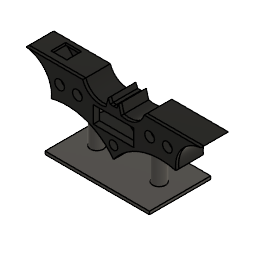
Bat Clock (Autodesk Fusion 360 design; units mm, degrees)
part number: 2025-11-05-17-47-18-195
part number: 2025-11-05-18-19-24-165
part number: 2025-11-05-18-19-49-827
part number: 2025-11-05-19-01-45-549
Autodesk Fusion 360 part; units mm, degrees
sketch "Sketch1" plane through (0, 0, 0) normal (0, 0, 1) x (1, 0, 0)
  line L0 (0, 0) -> (70.0024, 0)
  line L1 (0, 0) -> (0, -40.005)
  dimension "d1" = 70.0024
  dimension "d2" = 40.005
  constraint coincident L0.start L1.start
  constraint horizontal L0
  constraint perpendicular L0 L1
  measures "d1" distance of L0.start L0.end
  measures "d2" distance of L0.start L1.end
sketch "Sketch2" plane through (0, 0, 0) normal (0, 0, 1) x (1, 0, 0)
  line L0 (0, 0) -> (0, -40.64)
  arc A0 (0, -38.1) -> (-51.5436, -20.32) centre (-38.6745, -66.6145) ccw
  arc A1 (-51.5436, -20.32) -> (-72.3189, 6.443) centre (-75.1219, -17.178) ccw
  line L1 (-72.3189, 6.443) -> (-25.4, 6.443)
  arc A2 (-25.4, 6.443) -> (-6.3115, -3.5502) centre (-10.7993, 11.1049) ccw
  line L2 (-6.3115, -3.5502) -> (-4.3391, 3.8132)
  line L3 (-4.3391, 3.8132) -> (-2.7613, 0.1315)
  line L4 (-2.7613, 0.1315) -> (0, 0)
  arc A3 (51.5436, -20.32) -> (0, -38.1) centre (38.6745, -66.6145) ccw
  line L5 (4.3391, 3.8132) -> (2.7613, 0.1315)
  line L6 (72.3189, 6.443) -> (25.4, 6.443)
  arc A4 (6.3115, -3.5502) -> (25.4, 6.443) centre (10.7993, 11.1049) ccw
  line L7 (2.7613, 0.1315) -> (0, 0)
  arc A5 (72.3189, 6.443) -> (51.5436, -20.32) centre (75.1219, -17.178) ccw
  line L8 (6.3115, -3.5502) -> (4.3391, 3.8132)
  constraint coincident L0.start L4.end
  constraint vertical L0
  constraint coincident L0 A0.start
  constraint horizontal L1
  constraint symmetric L0 A0.start A3.end
  constraint symmetric L0 A0.end A3.start
  constraint symmetric L0 A0 A3
  constraint symmetric L0 A1.end L6.start
  constraint symmetric L0 A1 A5
  constraint symmetric L0 L1.end L6.end
  constraint symmetric L0 A2.end A4.start
  constraint symmetric L0 A2 A4
  constraint symmetric L0 L2.end L5.start
  constraint symmetric L0 L3.end L5.end
  constraint symmetric L0 L4.end L7.end
extrude "Extrude1" add sketch "Sketch2" along normal blind 20.32 makes body 1
shell "Shell1" thickness 2.032 removed faces 1 at (39.0183, -7.033, 20.32) on bodies 1
sketch "Sketch4" plane through (0, 0, 20.32) normal (0, 0, 1) x (-1, 0, 0)
  arc A0 (-60.9613, -4.411) -> (-49.308, 17.6745) centre (-75.1219, 17.178) ccw
  arc A1 (-49.308, 17.6745) -> (0, 34.795) centre (-38.6745, 66.6145) ccw
  arc A2 (0, 34.795) -> (49.308, 17.6745) centre (38.6745, 66.6145) ccw
  arc A3 (49.308, 17.6745) -> (60.9613, -4.411) centre (75.1219, 17.178) ccw
  line L0 (60.9613, -4.411) -> (26.8156, -4.411)
  arc A4 (26.8156, -4.411) -> (4.6283, 5.1201) centre (10.7993, -11.1049) ccw
  line L1 (4.6283, 5.1201) -> (3.7539, 1.8555)
  line L2 (3.7539, 1.8555) -> (0, 2.0343)
  line L3 (0, 2.0343) -> (-3.7539, 1.8555)
  line L4 (-3.7539, 1.8555) -> (-4.6283, 5.1201)
  arc A5 (-4.6283, 5.1201) -> (-26.8156, -4.411) centre (-10.7993, -11.1049) ccw
  line L5 (-26.8156, -4.411) -> (-60.9613, -4.411)
  line L6 (-72.3189, -6.443) -> (-25.4, -6.443)
  arc A6 (-6.3115, 3.5502) -> (-25.4, -6.443) centre (-10.7993, -11.1049) ccw
  line L7 (-6.3115, 3.5502) -> (-4.3391, -3.8132)
  line L8 (-4.3391, -3.8132) -> (-2.7613, -0.1315)
  line L9 (-2.7613, -0.1315) -> (0, 0)
  line L10 (0, 0) -> (2.7613, -0.1315)
  line L11 (2.7613, -0.1315) -> (4.3391, -3.8132)
  line L12 (4.3391, -3.8132) -> (6.3115, 3.5502)
  arc A7 (25.4, -6.443) -> (6.3115, 3.5502) centre (10.7993, -11.1049) ccw
  line L13 (25.4, -6.443) -> (72.3189, -6.443)
  arc A8 (51.5436, 20.32) -> (72.3189, -6.443) centre (75.1219, 17.178) ccw
  arc A9 (0, 38.1) -> (51.5436, 20.32) centre (38.6745, 66.6145) ccw
  arc A10 (-51.5436, 20.32) -> (0, 38.1) centre (-38.6745, 66.6145) ccw
  arc A11 (-72.3189, -6.443) -> (-51.5436, 20.32) centre (-75.1219, 17.178) ccw
sketch "Sketch5" plane through (0, 0, 20.32) normal (0, 0, 1) x (-1, 0, 0)
  arc A0 (-60.9613, -4.411) -> (-49.308, 17.6745) centre (-75.1219, 17.178) ccw
  arc A1 (-49.308, 17.6745) -> (0, 34.795) centre (-38.6745, 66.6145) ccw
  arc A2 (0, 34.795) -> (49.308, 17.6745) centre (38.6745, 66.6145) ccw
  arc A3 (49.308, 17.6745) -> (60.9613, -4.411) centre (75.1219, 17.178) ccw
  line L0 (60.9613, -4.411) -> (26.8156, -4.411)
  arc A4 (26.8156, -4.411) -> (4.6283, 5.1201) centre (10.7993, -11.1049) ccw
  line L1 (4.6283, 5.1201) -> (3.7539, 1.8555)
  line L2 (3.7539, 1.8555) -> (0, 2.0343)
  line L3 (0, 2.0343) -> (-3.7539, 1.8555)
  line L4 (-3.7539, 1.8555) -> (-4.6283, 5.1201)
  arc A5 (-4.6283, 5.1201) -> (-26.8156, -4.411) centre (-10.7993, -11.1049) ccw
  line L5 (-26.8156, -4.411) -> (-60.9613, -4.411)
  line L6 (-72.3189, -6.443) -> (-25.4, -6.443)
  arc A6 (-6.3115, 3.5502) -> (-25.4, -6.443) centre (-10.7993, -11.1049) ccw
  line L7 (-6.3115, 3.5502) -> (-4.3391, -3.8132)
  line L8 (-4.3391, -3.8132) -> (-2.7613, -0.1315)
  line L9 (-2.7613, -0.1315) -> (0, 0)
  line L10 (0, 0) -> (2.7613, -0.1315)
  line L11 (2.7613, -0.1315) -> (4.3391, -3.8132)
  line L12 (4.3391, -3.8132) -> (6.3115, 3.5502)
  arc A7 (25.4, -6.443) -> (6.3115, 3.5502) centre (10.7993, -11.1049) ccw
  line L13 (25.4, -6.443) -> (72.3189, -6.443)
  arc A8 (51.5436, 20.32) -> (72.3189, -6.443) centre (75.1219, 17.178) ccw
  arc A9 (0, 38.1) -> (51.5436, 20.32) centre (38.6745, 66.6145) ccw
  arc A10 (-51.5436, 20.32) -> (0, 38.1) centre (-38.6745, 66.6145) ccw
  arc A11 (-72.3189, -6.443) -> (-51.5436, 20.32) centre (-75.1219, 17.178) ccw
extrude "Extrude3" add sketch "Sketch5" against normal blind 2.54 separate body contours A0 A1 A2 A3 L0 A4 L1 L2 L3 L4 A5 L5 makes body 2
extrude "Extrude4" add sketch "Sketch5" along normal blind 2.54 contours A0 A1 A2 A3 L0 A4 L1 L2 L3 L4 A5 L5 | L6 A6 L7 L8 L9 L10 L11 L12 A7 L13 A8 A9 A10 A11 bodies 2
copy_body "Body->Comp1" bodies 1 removing the originals makes body 3 in component "Body"
copy_body "Body->Comp2" bodies 2 removing the originals makes body 4 in component "Lid"
sketch "Sketch6" plane through (0, 0, 46.2676) normal (0, 0, 1) x (-1, 0, 0)
  line L0 (-12.6934, 7.182) -> (-10.721, -0.1814)
  line L1 (-10.721, -0.1814) -> (-9.1432, 3.5003)
  line L2 (-9.1432, 3.5003) -> (-6.3819, 3.6318)
  line L3 (-6.3819, 3.6318) -> (-3.6206, 3.5003)
  line L4 (-3.6206, 3.5003) -> (-2.0428, -0.1814)
  line L5 (-2.0428, -0.1814) -> (-0.0704, 7.182)
  arc A0 (19.0181, -2.8112) -> (-0.0704, 7.182) centre (4.4174, -7.4731) ccw
  line L6 (19.0181, -2.8112) -> (65.937, -2.8112)
  arc A1 (45.1617, 23.9518) -> (65.937, -2.8112) centre (68.74, 20.8098) ccw
  arc A2 (-6.3819, 41.7318) -> (45.1617, 23.9518) centre (32.2926, 70.2463) ccw
  arc A3 (-57.9256, 23.9518) -> (-6.3819, 41.7318) centre (-45.0564, 70.2463) ccw
  arc A4 (-78.7008, -2.8112) -> (-57.9256, 23.9518) centre (-81.5038, 20.8098) ccw
  line L7 (-78.7008, -2.8112) -> (-31.7819, -2.8112)
  arc A5 (-12.6934, 7.182) -> (-31.7819, -2.8112) centre (-17.1813, -7.4731) ccw
  line L8 (-23.0838, 24.7751) -> (10.32, 24.7751)
  line L9 (10.32, 24.7751) -> (10.32, 10.785)
  line L10 (10.32, 10.785) -> (-23.0838, 10.785)
  line L11 (-23.0838, 10.785) -> (-23.0838, 24.7751)
  line L12 (-23.0838, 24.7751) -> (10.32, 10.785) construction
  line L13 (10.32, 24.7751) -> (-23.0838, 10.785) construction
  point P0 (-6.3819, 17.78)
  dimension "d14" = 58.42
  dimension "d15" = 58.42
  constraint horizontal L8
  constraint perpendicular L8 L9
  constraint parallel L8 L10
  constraint parallel L9 L11
  constraint coincident L12 P0
  constraint coincident L13 P0
  measures "d14" distance of A4.centre L11
  measures "d15" distance of A1.centre L9
extrude "Extrude1'" cut sketch "Sketch6" against normal blind 17.78 contours L8 L9 L10 L11 sketch seen with x (1, 0, 0) y (0, 1, 0) z (0, 0, 1) at (-6.3819, 3.6318, -23.4076) bodies 4 in component "Lid"
sketch "Sketch7" plane through (0, 0, 22.86) normal (0, 0, 1) x (-1, 0, 0)
  line L0 (16.7019, 21.1433) -> (16.7019, 7.1532)
  line L1 (16.7019, 7.1532) -> (-16.7019, 7.1532)
  line L2 (-16.7019, 7.1532) -> (-16.7019, 21.1433)
  line L3 (-16.7019, 21.1433) -> (16.7019, 21.1433)
  line L4 (-6.3115, 3.5502) -> (-4.3391, -3.8132)
  line L5 (-4.3391, -3.8132) -> (-2.7613, -0.1315)
  line L6 (-2.7613, -0.1315) -> (0, 0)
  line L7 (0, 0) -> (2.7613, -0.1315)
  line L8 (2.7613, -0.1315) -> (4.3391, -3.8132)
  line L9 (4.3391, -3.8132) -> (6.3115, 3.5502)
  arc A0 (25.4, -6.443) -> (6.3115, 3.5502) centre (10.7993, -11.1049) ccw
  line L10 (25.4, -6.443) -> (72.3189, -6.443)
  arc A1 (51.5436, 20.32) -> (72.3189, -6.443) centre (75.1219, 17.178) ccw
  arc A2 (0, 38.1) -> (51.5436, 20.32) centre (38.6745, 66.6145) ccw
  arc A3 (-51.5436, 20.32) -> (0, 38.1) centre (-38.6745, 66.6145) ccw
  arc A4 (-72.3189, -6.443) -> (-51.5436, 20.32) centre (-75.1219, 17.178) ccw
  line L11 (-72.3189, -6.443) -> (-25.4, -6.443)
  arc A5 (-6.3115, 3.5502) -> (-25.4, -6.443) centre (-10.7993, -11.1049) ccw
  circle A6 centre (44.5861, 6.8536) radius 4.0005
  line L12 (0, 0) -> (0, 45.72) construction
  circle A7 centre (29.8835, 6.8536) radius 4.0005
  line L13 (44.5861, 6.8536) -> (56.3321, 6.8536) construction
  line L14 (44.5861, 6.8536) -> (0, 7.1532) construction
  circle A8 centre (-29.8835, 6.8536) radius 4.0005
  circle A9 centre (-44.5861, 6.8536) radius 4.0005
  circle A10 centre (0, 27.94) radius 3.5052
  point P0 (-44.5861, 6.8536)
  point P1 (-44.5861, 6.8536)
  dimension "d22" = 8.001
  dimension "d23" = 7.0104
  constraint coincident L6.end L7.start
  constraint perpendicular L3 L12
  constraint equal A6 A7
  constraint coincident A6.centre L13.start
  constraint horizontal L13
  constraint midpoint L1 L14.end
  constraint horizontal A6.centre A7.centre
  constraint symmetric A6 L12 A9
  constraint symmetric L12 A7 A8
  constraint symmetric L12 A6.centre P1
  constraint coincident L12 A10.centre
  measures "d22" diameter of A6
  measures "d23" diameter of A10
extrude "Extrude2" cut sketch "Sketch7" against normal blind 10.16 contours A6 | A7 | A8 | A9 | A10 bodies 4 in component "Lid"
sketch "Sketch8" plane through (0, 6.443, 0) normal (0, 1, 0) x (-1, 0, 0)
  line L0 (25.4, 0) -> (72.3189, 0)
  line L1 (72.3189, 0) -> (72.3189, 20.32)
  line L2 (72.3189, 20.32) -> (25.4, 20.32)
  line L3 (25.4, 20.32) -> (25.4, 0)
  line L4 (46.1169, 15.3428) -> (59.1217, 15.3428)
  line L5 (59.1217, 15.3428) -> (59.1217, 3.354)
  line L6 (59.1217, 3.354) -> (46.1169, 3.354)
  line L7 (46.1169, 3.354) -> (46.1169, 15.3428)
  dimension "d26" = 13.0048
  dimension "d27" = 11.9888
  constraint horizontal L4
  constraint vertical L5
  constraint horizontal L6
  constraint vertical L7
  measures "d26" distance of L4.start L4.end
  measures "d27" distance of L4.start L6.end
extrude "Extrude1''" cut sketch "Sketch8" against normal blind 2.54 contours L4 L5 L6 L7 bodies 3 in component "Body"
sketch "Sketch9" plane through (0, 0, 0) normal (0, 0, 1) x (1, 0, 0)
  circle A0 centre (-10.4491, 0) radius 5.3128
  line L0 (-36.2174, 10.8533) -> (-36.2174, -9.4667)
  line L1 (15.3263, 10.8533) -> (15.3263, -9.4667) construction
  circle A1 centre (41.1016, 0) radius 5.3128
  point P0 (30.6526, 0)
  dimension "d30" = 25.7683
  dimension "d32" = 25.7753
  dimension "d33" = 51.5436
  constraint symmetric origin L1 P0
  constraint symmetric A0 L1 A1
  measures "d30" distance of A0.centre L0
  measures "d32" distance of A0.centre L1
  measures "d33" distance of L0 L1
extrude "Extrude2'" cut sketch "Sketch9" along normal blind 53.34 sketch seen with x (1, 0, 0) y (0, 0, -1) z (0, 1, 0) at (-15.3263, -69.8065, 10.8533) bodies 3 in component "Body"
extrude "Extrude5" add sketch "Sketch9" along normal blind 33.02 separate body makes body 5 at (46.388, -0.529, 11.0067) makes body 6 at (-5.1627, -0.529, 11.0067)
sketch "Sketch10" plane through (0, 0, 0) normal (0, 0, 1) x (1, 0, 0)
  line L0 (58.42, 25.4) -> (-27.94, 25.4)
  line L1 (-27.94, 25.4) -> (-27.94, -25.4)
  line L2 (-27.94, -25.4) -> (58.42, -25.4)
  line L3 (58.42, -25.4) -> (58.42, 25.4)
  line L4 (58.42, 25.4) -> (-27.94, -25.4) construction
  line L5 (-27.94, 25.4) -> (58.42, -25.4) construction
  point P0 (15.24, 0)
  constraint horizontal L0
  constraint perpendicular L0 L1
  constraint parallel L0 L2
  constraint parallel L1 L3
  constraint coincident L4 P0
  constraint coincident L5 P0
extrude "Extrude6" cut sketch "Sketch10" along normal blind 2.54 bodies 5 6
extrude "Extrude7" add sketch "Sketch10" along normal blind 2.54 bodies 5 6
copy_body "Body->Comp3" bodies 5 removing the originals makes body 7 in component "Stand"
component "Lid" placed x (1, 0, 0) y (0, 0, 1) z (0, -1, 0) at (15.3263, 10.8533, 49.4865)
component "Body" placed x (1, 0, 0) y (0, 0, 1) z (0, -1, 0) at (15.3263, 10.8533, 49.4865)
component "Stand" placed x (1, 0, 0) y (0, 1, 0) z (0, 0, 1) at (0, 0, 0)
